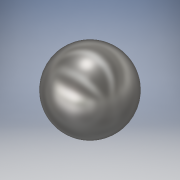
# Autodesk Inventor part: Bearings - Ball
Saved by Autodesk Inventor 2019 (Build 230136000, 136)
## iProperties
Created: 2020-12-03
Part Number: Bearings - Ball
Material: Stainless Steel
Document SubType Name: Modeling
Designer: Anass Hamdi
Density: 8 g/cm^3
Appearance: Semi-Polished
Author: Anass Hamdi
Autodesk Inventor part; units mm, degrees
ref_plane "YZ Plane" through (0, 0, 0) normal (1, 0, 0) x (0, 1, 0)
ref_plane "XZ Plane" through (0, 0, 0) normal (0, 1, 0) x (-1, 0, 0)
ref_plane "XY Plane" through (0, 0, 0) normal (0, 0, 1) x (1, 0, 0)
sketch "Sketch1" plane through (0, 0, 0) normal (0, 0, 1) x (1, 0, 0)
  arc A0 (0, -2) -> (0, 2) centre (0, 0) ccw
  line L0 (0, -2) -> (0, 2)
  line L1 (0, -2.8) -> (0, 2.8) projected
  dimension "d0" = 4
  constraints: 2 end point, 2 point on circle, 1 centre point, 1 coincident, 1 vertical
  measures "d0" diameter of A0
revolve "Revolution1" add sketch "Sketch1" angle 360 about axis through (0, -10, 0) along (0, 1, 0)
body "Solid1"
